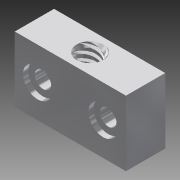
# Autodesk Inventor part: Metric ACME Block
Saved by Autodesk Inventor 2014 SP1 (Build 180222100, 222)
## iProperties
Created: 2016-04-10
Part Number: Metric ACME Block
Material: Generic
Document SubType Name: Modeling
Designer: Ben
Density: 1 g/cm^3
Appearance: Default
Author: Ben
Autodesk Inventor part; units mm, degrees
ref_plane "YZ Plane" through (0, 0, 0) normal (1, 0, 0) x (0, 1, 0)
ref_plane "XZ Plane" through (0, 0, 0) normal (0, 1, 0) x (-1, 0, 0)
ref_plane "XY Plane" through (0, 0, 0) normal (0, 0, 1) x (1, 0, 0)
sketch "Sketch1" plane through (0, 0, 0) normal (0, 0, 1) x (1, 0, 0)
  line L0 (-17, 10) -> (17, 10)
  line L1 (17, 10) -> (17, -10)
  line L2 (17, -10) -> (-17, -10)
  line L3 (-17, -10) -> (-17, 10)
  line L4 (0, 10) -> (0, -10) construction
  line L5 (-17, 0) -> (17, 0) construction
  point P0 (0, 0)
  dimension "d0" = 20
  dimension "d1" = 34
  constraints: 12 end point, 6 midpoint, 2 parallel, 1 horizontal, 1 perpendicular
  measures "d0" distance of L2.end L0.start
  measures "d1" distance of L0.start L0.end
extrude "Extrusion1" add sketch "Sketch1" along normal blind 12
sketch "Sketch2" plane through (-17, -10, 0) normal (0, -1, 0) x (1, 0, 0)
  circle A0 centre (17, 6) radius 3.1
  point P0 (17, 0)
  dimension "d4" = 6.2
  constraints: 1 centre point
  measures "d4" diameter of A0
extrude "Extrusion2" cut sketch "Sketch2" against normal up to next
sketch "Sketch3" plane through (0, 0, 12) normal (0, 0, 1) x (1, 0, 0)
  line L0 (17, 10) -> (-17, 10) projected
  line L1 (-17, 10) -> (-17, -10) projected
  line L2 (-17, -10) -> (17, -10) projected
  line L3 (17, -10) -> (17, 10) projected
  circle A0 centre (-10, 0) radius 2.525
  circle A1 centre (10, 0) radius 2.525
  line L4 (0, 10) -> (0, -10) construction
  line L5 (-17, 0) -> (17, 0) construction
  point P0 (0, 0)
  dimension "d7" = 5.05
  dimension "d8" = 5.05
  dimension "d9" = 20
  constraints: 4 end point, 4 midpoint, 2 centre point, 1 point on line, 1 symmetric about line
  measures "d7" diameter of A0
  measures "d8" diameter of A1
  measures "d9" distance of A1.centre A0.centre
extrude "Extrusion3" cut sketch "Sketch3" against normal up to next contours A0 | A1
sketch "Sketch4" plane through (0, 0, 12) normal (0, 0, 1) x (1, 0, 0)
  circle A0 centre (-10, 0) radius 2.525 projected
  circle A1 centre (10, 0) radius 2.525 projected
  circle A2 centre (-10, 0) radius 4.5
  circle A3 centre (10, 0) radius 4.5
  point P0 (0, 0)
  dimension "d12" = 9
  constraints: 2 centre point, 2 coincident, 1 equal radius
  measures "d12" diameter of A2
extrude "Extrusion4" cut sketch "Sketch4" against normal blind 1.6
sketch "Sketch5" plane through (0, 0, 0) normal (0, 0, -1) x (-1, 0, 0)
  circle A0 centre (10, 0) radius 2.525 projected
  circle A1 centre (-10, 0) radius 2.525 projected
  line L0 (-6, -2.3094) -> (-10, -4.6188)
  line L1 (-10, -4.6188) -> (-14, -2.3094)
  line L2 (-14, -2.3094) -> (-14, 2.3094)
  line L3 (-14, 2.3094) -> (-10, 4.6188)
  line L4 (-10, 4.6188) -> (-6, 2.3094)
  line L5 (-6, 2.3094) -> (-6, -2.3094)
  line L6 (14, -2.3094) -> (10, -4.6188)
  line L7 (10, -4.6188) -> (6, -2.3094)
  line L8 (6, -2.3094) -> (6, 2.3094)
  line L9 (6, 2.3094) -> (10, 4.6188)
  line L10 (10, 4.6188) -> (14, 2.3094)
  line L11 (14, 2.3094) -> (14, -2.3094)
  point P0 (0, 0)
  dimension "d15" = 8
  dimension "d16" = 8
  constraints: 24 end point, 2 coincident, 26 other
  measures "d15" distance between parallel lines of L5 L2
  measures "d16" distance between parallel lines of L11 L8
extrude "Extrusion5" cut sketch "Sketch5" against normal blind 4.97
sketch "Sketch7" plane through (0, 0, 0) normal (1, 0, 0) x (0, 1, 0)
  line L0 (-10, 0) -> (10, 0) projected
  line L1 (-10, 0) -> (-10, 12) projected
  line L2 (10, 12) -> (-10, 12) projected
  line L3 (10, 0) -> (10, 12) projected
  line L4 (-10, 9.1) -> (10, 9.1) projected
  line L5 (10, 6) -> (15.5091, 6)
  line L6 (10, 9.1) -> (10.2679, 10.1)
  line L7 (10, 9.1) -> (11.0353, 9.1) construction
  line L8 (10.2679, 10.1) -> (10.8321, 10.1)
  line L9 (10.8321, 10.1) -> (11.1, 9.1)
  line L10 (11.1, 9.1) -> (12, 9.1)
  line L11 (10, 9.1) -> (11.1, 9.1)
  line L12 (12, 9.1) -> (12.2679, 10.1)
  line L13 (12, 9.1) -> (13.0353, 9.1) construction
  line L14 (12.2679, 10.1) -> (12.8321, 10.1)
  line L15 (12.8321, 10.1) -> (13.1, 9.1)
  line L16 (13.1, 9.1) -> (14, 9.1)
  line L17 (12, 9.1) -> (13.1, 9.1)
  line L18 (14, 9.1) -> (14.2679, 10.1)
  line L19 (14, 9.1) -> (15.0353, 9.1) construction
  line L20 (14.2679, 10.1) -> (14.8321, 10.1)
  line L21 (14.8321, 10.1) -> (15.1, 9.1)
  line L22 (15.1, 9.1) -> (16, 9.1)
  line L23 (14, 9.1) -> (15.1, 9.1)
  line L24 (16, 9.1) -> (16.2679, 10.1)
  line L25 (16, 9.1) -> (17.0353, 9.1) construction
  line L26 (16.2679, 10.1) -> (16.8321, 10.1)
  line L27 (16.8321, 10.1) -> (17.1, 9.1)
  line L28 (17.1, 9.1) -> (18, 9.1)
  line L29 (16, 9.1) -> (17.1, 9.1)
  point P0 (0, 0)
  dimension "d25" = 75
  dimension "d26" = 30
  dimension "d28" = 4.1
  dimension "d29" = 1.1
  dimension "d30" = 2
  dimension "d33" = 2
  constraints: 50 end point, 2 collinear, 2 horizontal, 2 parallel, 1 equal length, 1 midpoint, 1 perpendicular, 36 other
  measures "d25" angle of L7 L6
  measures "d26" angle of L9 L6
  measures "d28" distance from line of L5 L6.end
  measures "d29" distance from line of L9.end L3
  measures "d30" distance from line of L10.end L3
  measures "d33" distance of L4.end L17.start
chamfer "Chamfer1" distance 1 angle 45 2 edges at (-3.1, -10, 6) (-3.1, 10, 6)
coil "Coil2" sketch "Sketch7" operation cut axis through (0, 10, 6) along (0, -1, 0) pitch 8 turns 3.5 hand right contours L24 L26 L27 L29 | L18 L20 L21 L23 | L12 L14 L15 L17 | L6 L8 L9 L11
body "Solid1"
